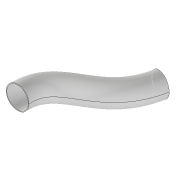
# Autodesk Inventor part: Rohr_1
Saved by Autodesk Inventor 2020 (Build 240168000, 168)
## iProperties
Created: 2020-04-08
Part Number: Rohr_1
Material: Generisch
Document SubType Name: Modeling
Designer: franz
Density: 1 g/cm^3
Appearance: Vorgabe
Author: franz
Autodesk Inventor part; units mm, degrees
ref_plane "YZ Plane" through (0, 0, 0) normal (1, 0, 0) x (0, 1, 0)
ref_plane "XZ Plane" through (0, 0, 0) normal (0, 1, 0) x (-1, 0, 0)
ref_plane "XY Plane" through (0, 0, 0) normal (0, 0, 1) x (1, 0, 0)
sketch "Skizze1" plane through (0, 0, 0) normal (0, 0, 1) x (1, 0, 0)
  circle A0 centre (0, 0) radius 85
  circle A1 centre (0, 0) radius 90
  dimension "d0" = 170
  dimension "d1" = 180
  constraints: 2 centre point, 2 coincident
  measures "d0" diameter of A0
  measures "d1" diameter of A1
sketch "Skizze2" plane through (0, 0, 0) normal (0, 1, 0) x (-1, 0, 0)
  spline S0 degree 4 poles (0, 0) (121.0567, -287.7751) (-72.7639, -359.3504) (9.2278, -553.12) (7.5368, -697.2955) knots 0 0 0 0 0 1 1 1 1 1
  line L0 (8.3346, -629.2733) -> (6.7389, -765.3176) construction
  arc A0 (2.4963, -750.9318) -> (3.7557, -643.5556) centre (-321.4192, -693.4372) ccw construction
  point P0 (18.675, -324.7179)
  point P1 (-4.4975, -511.6538)
  constraints: 2 end point, 2 midpoint, 1 centre point, 1 point on circle, 6 other
sweep "Sweeping1" add profiles "Skizze1" path "Skizze2"
